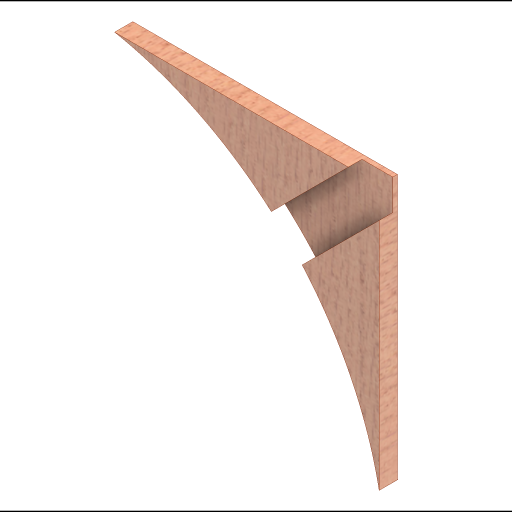
# Autodesk Inventor part: Wind Tunnel Fan Shroud Corner Mod Strap
Saved by Autodesk Inventor 2023 (Build 270158000, 158)
## iProperties
Created: 2022-01-23
Part Number: Wind Tunnel Fan Shroud Corner Mod Strap
Material: Wood (Oak)
Document SubType Name: Modeling
Designer: kamer
Density: 0.76 g/cm^3
Appearance: White Oak - Natural Medium Gloss
Author: kamer
Autodesk Inventor part; units mm, degrees
ref_plane "YZ Plane" through (0, 0, 0) normal (1, 0, 0) x (0, 1, 0)
ref_plane "XZ Plane" through (0, 0, 0) normal (0, 1, 0) x (-1, 0, 0)
ref_plane "XY Plane" through (0, 0, 0) normal (0, 0, 1) x (1, 0, 0)
sketch "Sketch1" plane through (0, 0, 0) normal (0, 0, 1) x (1, 0, 0)
  circle A0 centre (0, 0) radius 215.9
  line L0 (-215.9, 215.9) -> (215.9, 215.9)
  line L1 (215.9, 215.9) -> (215.9, -215.9)
  line L2 (215.9, -215.9) -> (-215.9, -215.9)
  line L3 (-215.9, -215.9) -> (-215.9, 215.9)
  point P0 (215.9, 0)
  point P1 (0, 215.9)
  dimension "d0" = 431.8
  dimension "d1" = 431.8
  dimension "d2" = 431.8
  dimension "d3" = 215.9
  dimension "d4" = 215.9
  constraints: 8 end point, 2 parallel, 1 centre point, 1 coincident, 1 horizontal, 1 perpendicular
  measures "d0" diameter of A0
  measures "d1" distance of L1.end L2.end
  measures "d2" distance of L0.end L1.end
  measures "d3" distance from line of L3 point (0, 0)
  measures "d4" distance from line of L0 point (0, 0)
extrude "Extrusion1" add sketch "Sketch1" along normal blind 11.938 contours A0 L0 L1
sketch "Sketch2" plane through (0, 0, 11.938) normal (0, 0, 1) x (1, 0, 0)
  circle A0 centre (0, 0) radius 220
  dimension "d7" = 440
  constraints: 1 centre point, 1 coincident
  measures "d7" diameter of A0
extrude "Extrusion2" cut sketch "Sketch2" against normal through all
sketch "Sketch3" plane through (0, 0, 11.938) normal (0, 0, 1) x (1, 0, 0)
  line L0 (215.9, 215.9) -> (42.2752, 215.9) projected
  line L1 (215.9, 215.9) -> (197.9422, 215.9)
  line L2 (215.9, 42.2752) -> (215.9, 215.9) projected
  line L3 (215.9, 215.9) -> (215.9, 197.9368)
  line L4 (215.9, 197.9368) -> (135.0791, 117.1158)
  line L5 (135.0791, 117.1158) -> (117.1185, 135.0763)
  line L6 (117.1185, 135.0763) -> (197.9422, 215.9)
  point P0 (0, 0)
  dimension "d10" = 25.4
  dimension "d11" = 135
  dimension "d12" = 135
  dimension "d13" = 17.9578
  dimension "d14" = 90
  dimension "d15" = 127
  constraints: 10 end point, 2 point on line
  measures "d10" distance of L3.end L1.end
  measures "d11" angle of L0 L6
  measures "d12" angle of L4 L2
  measures "d13" distance of L0.start L1.end
  measures "d14" angle of L5 L6
  measures "d15" distance from line of L0.start L5
extrude "Extrusion3" cut sketch "Sketch3" against normal blind 8.89
sketch "Sketch5" plane through (0, 0, 11.938) normal (0, 0, 1) x (1, 0, 0)
  arc A0 (164.2856, 146.3224) -> (146.3253, 164.2831) centre (0, 0) ccw projected
  line L0 (215.9, 197.9368) -> (164.2856, 146.3224) projected
  line L1 (215.9, 215.9) -> (215.9, 197.9368) projected
  line L2 (197.9422, 215.9) -> (215.9, 215.9) projected
  line L3 (146.3253, 164.2831) -> (197.9422, 215.9) projected
  line L4 (137.2766, 157.4974) -> (211.5205, 231.7413)
  line L5 (211.5205, 231.7413) -> (233.2717, 213.0454)
  line L6 (233.2717, 213.0454) -> (157.5001, 137.2738)
  line L7 (157.5001, 137.2738) -> (137.2766, 157.4974)
  dimension "d22" = 90
  dimension "d25" = 4.32
  dimension "d26" = 1.6002
  dimension "d27" = 1.6002
  constraints: 8 end point
  measures "d22" angle of L7 L4
  measures "d25" angle of L7 L5
  measures "d26" distance between parallel lines of L4 L3
  measures "d27" distance between parallel lines of L0 L6
extrude "Extrusion5" cut sketch "Sketch5" against normal up to surface (8.89 mm away) contours A0 L3 L2 L1 L0 | L4 L5 L6 L7
body "Solid1"
